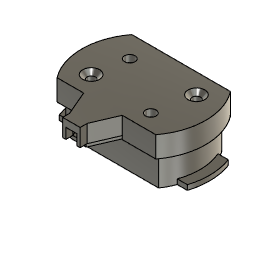
case (Autodesk Fusion 360 design; units mm, degrees)
Autodesk Fusion 360 part; units mm, degrees
sketch "Sketch1" plane through (0, 0, 0) normal (0, 0, 1) x (1, 0, 0)
  circle A0 centre (0, 0) radius 18.75
  line L0 (-17.5873, 6.5) -> (17.5873, 6.5)
  line L1 (-17.5873, -6.5) -> (17.5873, -6.5)
  circle A1 centre (0, 0) radius 16
  line L2 (-17.9252, 5.5) -> (-15.025, 5.5)
  line L3 (15.025, -5.5) -> (17.9252, -5.5)
  line L4 (-13.2288, -9) -> (13.2288, -9)
  line L5 (-13.2288, 9) -> (13.2288, 9)
  dimension "d1" = 37.5
  dimension "d2" = 13
  dimension "d17" = 32
  dimension "d18" = 1
  dimension "d19" = 1
  dimension "d20" = 18
  constraint coincident A0.centre A1.centre
  constraint coincident A0 L0.start
  constraint coincident A0 L0.end
  constraint horizontal L0
  constraint coincident A0 L1.start
  constraint coincident A0 L1.end
  constraint parallel L0 L1
  constraint vertical L0.start L1.start
  constraint concentric A0 A1
  constraint coincident A0 L2.start
  constraint coincident A1 L2.end
  constraint horizontal L2
  constraint coincident A1 L3.start
  constraint coincident A0 L3.end
  constraint parallel L2 L3
  constraint coincident A1 L4.start
  constraint coincident A1 L4.end
  constraint horizontal L4
  constraint coincident A1 L5.start
  constraint coincident A1 L5.end
  constraint parallel L0 L5
  constraint vertical L4.start L5.start
  measures "d1" diameter of A0
  measures "d2" distance of L0.end L1.end
  measures "d17" diameter of A1
  measures "d18" distance of L0 L2
  measures "d19" distance of L1 L3
  measures "d20" distance of L4 L5
extrude "Extrude1" add sketch "Sketch1" along normal blind 1.4 contours A0 L0 A1 L3 | L0 L1 A1 | L0 A1 L5 | A0 L1 A1 L2 | L1 A1 L4 makes body 1
sketch "Sketch2" plane through (0, 0, 0) normal (0, 0, -1) x (1, 0, 0)
  line L0 (-14.6202, 6.5) -> (-17.5873, 6.5)
  circle A0 centre (0, 0) radius 4.75
  circle A1 centre (0, 0) radius 7
  line L1 (4.75, 0) -> (7, 0)
  line L2 (4.4635, -1.6246) -> (6.5778, -2.3941)
  line L3 (4.4635, -1.6246) -> (0, 0)
  arc A2 (17.5873, -6.5) -> (17.9252, 5.5) centre (0, 0) ccw
  line L4 (14.6202, -6.5) -> (17.5873, -6.5)
  arc A3 (-15.025, -5.5) -> (-13.2288, -9) centre (0, 0) ccw
  line L5 (-13.2288, -9) -> (13.2288, -9)
  arc A4 (13.2288, -9) -> (14.6202, -6.5) centre (0, 0) ccw
  line L6 (17.9252, 5.5) -> (15.025, 5.5)
  arc A5 (15.025, 5.5) -> (13.2288, 9) centre (0, 0) ccw
  line L7 (13.2288, 9) -> (-13.2288, 9)
  arc A6 (-13.2288, 9) -> (-14.6202, 6.5) centre (0, 0) ccw
  arc A7 (-17.5873, 6.5) -> (-17.9252, -5.5) centre (0, 0) ccw
  line L8 (-17.9252, -5.5) -> (-15.025, -5.5)
  dimension "d10" = 9.5
  dimension "d11" = 14
  dimension "d12" = 20
  constraint coincident A0.centre A1.centre
  constraint coincident A0 L1.start
  constraint coincident A1 L1.end
  constraint horizontal L1
  constraint coincident A0 L2.start
  constraint coincident A1 L2.end
  constraint horizontal A0.centre L1.start
  constraint parallel L2 L3
  measures "d10" diameter of A0
  measures "d11" diameter of A1
  measures "d12" angle of L1 L2
extrude "Extrude2" add sketch "Sketch2" along normal blind 2.5 contours A0 | A0 A1 L1 L2 picked at (6.2235, -0.4547) bodies 1
sketch "Sketch4" plane through (0, 0, 1.4) normal (0, 0, 1) x (-1, 0, 0)
  arc A0 (13.2288, -9) -> (15.025, -5.5) centre (0, 0) ccw
  line L0 (15.025, -5.5) -> (17.9252, -5.5)
  arc A1 (17.9252, -5.5) -> (17.5873, 6.5) centre (0, 0) ccw
  line L1 (17.5873, 6.5) -> (14.6202, 6.5)
  arc A2 (14.6202, 6.5) -> (13.2288, 9) centre (0, 0) ccw
  line L2 (13.2288, 9) -> (-13.2288, 9)
  arc A3 (-13.2288, 9) -> (-15.025, 5.5) centre (0, 0) ccw
  line L3 (-15.025, 5.5) -> (-17.9252, 5.5)
  arc A4 (-17.9252, 5.5) -> (-17.5873, -6.5) centre (0, 0) ccw
  line L4 (-17.5873, -6.5) -> (-14.6202, -6.5)
  arc A5 (-14.6202, -6.5) -> (-13.2288, -9) centre (0, 0) ccw
  line L5 (-13.2288, -9) -> (13.2288, -9)
  circle A6 centre (0, 0) radius 16
  constraint coincident A0.centre A1.centre
  constraint tangent A0 A6
extrude "Extrude3" add sketch "Sketch4" along normal blind 8 contours A0 A2 L2 A3 A5 L5 A6 bodies 1
sketch "Sketch5" plane through (0, 0, 0) normal (0, 0, -1) x (1, 0, 0)
  line L0 (4.75, 0) -> (7, 0)
  arc A0 (6.5778, -2.3941) -> (7, 0) centre (0, 0) ccw
  line L1 (6.5778, -2.3941) -> (4.4635, -1.6246)
  arc A1 (4.75, 0) -> (4.4635, -1.6246) centre (0, 0) ccw
  arc A2 (-15.025, -5.5) -> (-13.2288, -9) centre (0, 0) ccw
  line L2 (-13.2288, -9) -> (13.2288, -9)
  arc A3 (13.2288, -9) -> (14.6202, -6.5) centre (0, 0) ccw
  line L3 (14.6202, -6.5) -> (17.5873, -6.5)
  arc A4 (17.5873, -6.5) -> (17.9252, 5.5) centre (0, 0) ccw
  line L4 (17.9252, 5.5) -> (15.025, 5.5)
  arc A5 (15.025, 5.5) -> (13.2288, 9) centre (0, 0) ccw
  line L5 (13.2288, 9) -> (-13.2288, 9)
  arc A6 (-13.2288, 9) -> (-14.6202, 6.5) centre (0, 0) ccw
  line L6 (-14.6202, 6.5) -> (-17.5873, 6.5)
  arc A7 (-17.5873, 6.5) -> (-17.9252, -5.5) centre (0, 0) ccw
  line L7 (-17.9252, -5.5) -> (-15.025, -5.5)
  circle A8 centre (-12.5, 0) radius 2.75
  circle A9 centre (12.5, 0) radius 2.75
  line L8 (-12.5, 0) -> (12.5, 0)
  dimension "d23" = 5.5
  dimension "d24" = 5.5
  dimension "d25" = 25
  constraint coincident A8.centre L8.start
  constraint coincident A9.centre L8.end
  constraint midpoint L8 A0.centre
  constraint horizontal L8
  constraint coincident A0.centre A1.centre
  measures "d23" diameter of A8
  measures "d24" diameter of A9
  measures "d25" horizontal distance of A8.centre A9.centre
extrude "Extrude4" cut sketch "Sketch5" against normal blind 10 contours A8 | A9 bodies 1
sketch "Sketch6" plane through (0, 0, 9.4) normal (0, 0, 1) x (-1, 0, 0)
  circle A0 centre (12.5, 0) radius 2.75
  circle A1 centre (-12.5, 0) radius 2.75
  arc A2 (13.2288, -9) -> (13.2288, 9) centre (0, 0) ccw
  line L0 (13.2288, 9) -> (-13.2288, 9)
  arc A3 (-13.2288, 9) -> (-13.2288, -9) centre (0, 0) ccw
  line L1 (-13.2288, -9) -> (13.2288, -9)
  circle A4 centre (12.5, 0) radius 3.1
  circle A5 centre (-12.5, 0) radius 3.1
  dimension "d28" = 6.2
  dimension "d29" = 6.2
  constraint concentric A0 A4
  constraint concentric A1 A5
  measures "d28" diameter of A4
  measures "d29" diameter of A5
extrude "Extrude5" cut sketch "Sketch6" against normal blind 1.5 contours A4 | A5 bodies 1
sketch "Sketch7" plane through (0, 0, 9.4) normal (0, 0, 1) x (-1, 0, 0)
  circle A0 centre (-12.5, 0) radius 3.1
  circle A1 centre (12.5, 0) radius 3.1
  arc A2 (13.2288, -9) -> (13.2288, 9) centre (0, 0) ccw
  line L0 (13.2288, 9) -> (-13.2288, 9)
  arc A3 (-13.2288, 9) -> (-13.2288, -9) centre (0, 0) ccw
  line L1 (-13.2288, -9) -> (13.2288, -9)
  circle A4 centre (10, 5) radius 0.925
  circle A5 centre (-10, -5) radius 0.925
  line L2 (10, 5) -> (-10, -5)
  dimension "d32" = 1.85
  dimension "d33" = 1.85
  dimension "d34" = 20
  dimension "d35" = 10
  constraint coincident A4.centre L2.start
  constraint coincident A5.centre L2.end
  constraint midpoint L2 A2.centre
  constraint coincident A2.centre A3.centre
  measures "d32" diameter of A4
  measures "d33" diameter of A5
  measures "d34" horizontal distance of A4.centre A5.centre
  measures "d35" vertical distance of A4.centre A5.centre
extrude "Extrude6" cut sketch "Sketch7" against normal blind 8 contours A4 | A5 bodies 1
chamfer "Chamfer1" distance 0.3 angle 45 2 edges at (-9.1376, -5.3345, 9.4) (10.8624, 4.6655, 9.4) on bodies 1
copy_body "Body->Comp1" bodies 1 removing the originals makes body 2 in component "bottom"
sketch "Sketch3" plane through (0, 0, 9.4) normal (0, 0, 1) x (-1, 0, 0) in component "top"
  circle A0 centre (10, 5) radius 1.225
  circle A1 centre (-12.5, 0) radius 3.1
  circle A2 centre (12.5, 0) radius 3.1
  arc A3 (13.2288, -9) -> (13.2288, 9) centre (0, 0) ccw
  line L0 (13.2288, 9) -> (-13.2288, 9)
  arc A4 (-13.2288, 9) -> (-13.2288, -9) centre (0, 0) ccw
  line L1 (-13.2288, -9) -> (13.2288, -9)
  circle A5 centre (-10, -5) radius 1.225
  arc A6 (-13.4387, 9.4) -> (-13.4387, -9.4) centre (0, 0) ccw
  line L2 (-13.4387, -9.4) -> (13.4387, -9.4)
  arc A7 (13.4387, -9.4) -> (13.4387, 9.4) centre (0, 0) ccw
  line L3 (13.4387, 9.4) -> (-13.4387, 9.4)
  arc A8 (-14.0748, 10.65) -> (-14.0748, -10.65) centre (0, 0) ccw
  line L4 (-14.0748, -10.65) -> (14.0748, -10.65)
  arc A9 (14.0748, -10.65) -> (14.0748, 10.65) centre (0, 0) ccw
  line L5 (14.0748, 10.65) -> (-14.0748, 10.65)
  dimension "d41" = 0.4
  dimension "d42" = 1.65
extrude "Extrude1'" add sketch "Sketch3" along normal blind 3 and the other way blind 1 separate body contours A8 L4 A9 L5 makes body 3 in component "top"
sketch "Sketch4 (2)" plane through (0, 0, 12.4) normal (0, 0, 1) x (-1, 0, 0) in component "top"
  line L0 (-13.4387, 9.4) -> (13.4387, 9.4)
  arc A0 (13.4387, -9.4) -> (13.4387, 9.4) centre (0, 0) ccw
  line L1 (13.4387, -9.4) -> (-13.4387, -9.4)
  arc A1 (-13.4387, 9.4) -> (-13.4387, -9.4) centre (0, 0) ccw
  line L2 (14.0748, 10.65) -> (-14.0748, 10.65)
  arc A2 (-14.0748, 10.65) -> (-14.0748, -10.65) centre (0, 0) ccw
  line L3 (-14.0748, -10.65) -> (14.0748, -10.65)
  arc A3 (14.0748, -10.65) -> (14.0748, 10.65) centre (0, 0) ccw
extrude "Extrude2'" add sketch "Sketch4 (2)" along normal blind 2 contours L0 A0 L1 A1 | L2 A2 L3 A3 bodies 3 in component "top"
sketch "Sketch5 (2)" plane through (0, 0, 12.4) normal (0, 0, -1) x (1, 0, 0) in component "top"
  arc A0 (13.4387, -9.4) -> (13.4387, 9.4) centre (0, 0) ccw
  line L0 (13.4387, 9.4) -> (-13.4387, 9.4)
  arc A1 (-13.4387, 9.4) -> (-13.4387, -9.4) centre (0, 0) ccw
  line L1 (-13.4387, -9.4) -> (13.4387, -9.4)
  circle A2 centre (-10, 5) radius 1.2
  circle A3 centre (10, -5) radius 1.2
  line L2 (-10, 5) -> (10, -5)
  dimension "d49" = 2.4
  dimension "d50" = 2.4
  dimension "d51" = 20
  dimension "d52" = 10
  constraint coincident A2.centre L2.start
  constraint coincident A3.centre L2.end
  constraint midpoint L2 A0.centre
  constraint coincident A0.centre A1.centre
  measures "d49" diameter of A2
  measures "d50" diameter of A3
  measures "d51" horizontal distance of A2.centre A3.centre
  measures "d52" vertical distance of A2.centre A3.centre
extrude "Extrude3'" cut sketch "Sketch5 (2)" against normal blind 5 contours A2 | A3 bodies 3 in component "top"
sketch "Sketch6 (2)" plane through (0, 0, 12.4) normal (0, 0, -1) x (1, 0, 0) in component "top"
  circle A0 centre (-10, 5) radius 1.2
  circle A1 centre (10, -5) radius 1.2
  arc A2 (13.4387, -9.4) -> (13.4387, 9.4) centre (0, 0) ccw
  line L0 (13.4387, 9.4) -> (-13.4387, 9.4)
  arc A3 (-13.4387, 9.4) -> (-13.4387, -9.4) centre (0, 0) ccw
  line L1 (-13.4387, -9.4) -> (13.4387, -9.4)
  circle A4 centre (-10, 5) radius 1.2
  circle A5 centre (-10, 5) radius 2.7
  circle A6 centre (10, -5) radius 1.2
  circle A7 centre (10, -5) radius 2.7
  circle A8 centre (10, -5) radius 1.2
  dimension "d55" = 1.5
  dimension "d56" = 1.5
  constraint concentric A0 A4
  constraint concentric A0 A5
  constraint concentric A1 A6
  constraint concentric A6 A7
  constraint equal A0 A4
  constraint equal A6 A8
  measures "d55" distance of A4 A5
  measures "d56" distance of A6 A7
extrude "Extrude4'" add sketch "Sketch6 (2)" along normal blind 2 contours A5 | A7 bodies 3 in component "top"
chamfer "Chamfer1'" distance 1.2 angle 45 2 edges at (-11.1188, -4.5661, 14.4) (8.8812, 5.4339, 14.4) on bodies 3 in component "top"
sketch "Sketch8" plane through (0, 0, 14.4) normal (0, 0, 1) x (-1, 0, 0)
  circle A0 centre (10, 5) radius 2.4
  arc A1 (14.0748, -10.65) -> (14.0748, 10.65) centre (0, 0) ccw
  line L0 (14.0748, 10.65) -> (-14.0748, 10.65)
  arc A2 (-14.0748, 10.65) -> (-14.0748, -10.65) centre (0, 0) ccw
  line L1 (-14.0748, -10.65) -> (14.0748, -10.65)
  circle A3 centre (-10, -5) radius 2.4
  line L2 (6.5, 10.65) -> (3.5, 17.65)
  line L3 (3.5, 17.65) -> (-1.5, 17.65)
  line L4 (-1.5, 17.65) -> (-4.5, 10.65)
  point P0 (1, 17.65)
  dimension "d60" = 7
  dimension "d61" = 3
  dimension "d62" = 5
  dimension "d63" = 3
  dimension "d64" = 9
  constraint coincident L0 L2.start
  constraint parallel L0 L3
  constraint coincident L0 L4.end
  constraint midpoint L3 P0
  measures "d60" distance of L0 L3
  measures "d61" horizontal distance of L3.end L4.end
  measures "d62" distance of L2.end L3.end
  measures "d63" horizontal distance of L2.start L2.end
  measures "d64" horizontal distance of A0.centre P0
extrude "Extrude5'" add sketch "Sketch8" against normal blind 2 contours L0 L2 L3 L4 bodies 3 in component "top"
sketch "Sketch9" plane through (0, 0, 8.4) normal (0, 0, -1) x (1, 0, 0)
  line L0 (-13.4387, 9.4) -> (13.4387, 9.4)
  arc A0 (13.4387, -9.4) -> (13.4387, 9.4) centre (0, 0) ccw
  line L1 (13.4387, -9.4) -> (-13.4387, -9.4)
  arc A1 (-13.4387, 9.4) -> (-13.4387, -9.4) centre (0, 0) ccw
  line L2 (14.0748, 10.65) -> (-14.0748, 10.65)
  arc A2 (-14.0748, 10.65) -> (-14.0748, -10.65) centre (0, 0) ccw
  line L3 (-14.0748, -10.65) -> (14.0748, -10.65)
  arc A3 (14.0748, -10.65) -> (14.0748, 10.65) centre (0, 0) ccw
  line L4 (-6.5, 10.65) -> (-7.0357, 9.4)
  line L5 (4.5, 10.65) -> (5.0357, 9.4)
  line L6 (-3.5, 17.65) -> (-6.5, 10.65)
  line L7 (4.5, 10.65) -> (1.5, 17.65)
  constraint coincident L2 L4.start
  constraint coincident L0 L4.end
  constraint coincident L2 L5.start
  constraint coincident L0 L5.end
  constraint parallel L4 L6
  constraint parallel L5 L7
  constraint coincident L4.start L6.end
  constraint coincident L5.start L7.start
extrude "Extrude6'" cut sketch "Sketch9" against normal blind 4 contours L0 L2 L4 L5 bodies 3 in component "top"
sketch "Sketch10" plane through (0, 0, 12.4) normal (0, 0, -1) x (1, 0, 0)
  circle A0 centre (-10, 5) radius 2.7
  circle A1 centre (10, -5) radius 2.7
  line L0 (-3.5, 17.65) -> (-6.5, 10.65)
  line L1 (-6.5, 10.65) -> (-7.0357, 9.4)
  line L2 (-7.0357, 9.4) -> (-13.4387, 9.4)
  arc A2 (-13.4387, 9.4) -> (-13.4387, -9.4) centre (0, 0) ccw
  line L3 (-13.4387, -9.4) -> (13.4387, -9.4)
  arc A3 (13.4387, -9.4) -> (13.4387, 9.4) centre (0, 0) ccw
  line L4 (13.4387, 9.4) -> (5.0357, 9.4)
  line L5 (5.0357, 9.4) -> (4.5, 10.65)
  line L6 (4.5, 10.65) -> (1.5, 17.65)
  line L7 (1.5, 17.65) -> (-3.5, 17.65)
  line L8 (-7.0357, 9.4) -> (-6.1109, 9.4)
  line L9 (-6.1109, 9.4) -> (-2.5752, 17.65)
  line L10 (0.5752, 17.65) -> (4.1109, 9.4)
  line L11 (4.1109, 9.4) -> (5.0357, 9.4)
  dimension "d69" = 0.85
  dimension "d70" = 0.85
  constraint coincident L1.end L2.start
  constraint parallel L2 L8
  constraint coincident L7 L9.end
  constraint coincident L7 L10.start
  constraint coincident L4.end L5.start
  constraint parallel L4 L11
  constraint parallel L0 L9
  constraint parallel L6 L10
  measures "d69" distance of L0 L9
  measures "d70" distance of L6 L10
extrude "Extrude7" add sketch "Sketch10" along normal blind 3 contours L0 L1 L7 L8 L9 | L5 L6 L7 L10 L11 bodies 3 in component "top"
extrude "Extrude8" add 1 faces at (-0.4749, -17.65, 13.7333) along direction (0, -1, 0) blind 2 on bodies 3 bodies 3 in component "top"
sketch "Sketch11" plane through (0, 0, 14.4) normal (0, 0, 1) x (-1, 0, 0)
  circle A0 centre (10, 5) radius 2.4
  arc A1 (14.0748, -10.65) -> (14.0748, 10.65) centre (0, 0) ccw
  line L0 (14.0748, 10.65) -> (6.5, 10.65)
  line L1 (6.5, 10.65) -> (3.5, 17.65)
  line L2 (3.5, 17.65) -> (3.5, 19.65)
  line L3 (3.5, 19.65) -> (-1.5, 19.65)
  line L4 (-1.5, 19.65) -> (-1.5, 17.65)
  line L5 (-1.5, 17.65) -> (-4.5, 10.65)
  line L6 (-4.5, 10.65) -> (-14.0748, 10.65)
  arc A2 (-14.0748, 10.65) -> (-14.0748, -10.65) centre (0, 0) ccw
  line L7 (-14.0748, -10.65) -> (14.0748, -10.65)
  circle A3 centre (-10, -5) radius 2.4
  circle A4 centre (8.4, -4.4) radius 1.5
  circle A5 centre (-8, 6) radius 1.5
  circle A6 centre (10, 5) radius 1.2
  circle A7 centre (-10, -5) radius 1.2
  dimension "d75" = 3
  dimension "d76" = 3
  dimension "d77" = 1.6
  dimension "d78" = 0.6
  dimension "d79" = 2
  dimension "d80" = 1
  measures "d75" diameter of A4
  measures "d76" diameter of A5
  measures "d77" horizontal distance of A4.centre A0.centre
  measures "d78" vertical distance of A4.centre A3.centre
  measures "d79" horizontal distance of A5.centre A3.centre
  measures "d80" vertical distance of A5.centre A0.centre
extrude "Extrude9" cut sketch "Sketch11" against normal blind 2 contours A4 | A5 bodies 3 in component "top"
sketch "Sketch12" plane through (0, 0, 9.4) normal (0, 0, 1) x (-1, 0, 0)
  circle A0 centre (10, 5) radius 1.225
  circle A1 centre (-12.5, 0) radius 3.1
  circle A2 centre (12.5, 0) radius 3.1
  arc A3 (13.2288, -9) -> (13.2288, 9) centre (0, 0) ccw
  line L0 (13.2288, 9) -> (-13.2288, 9)
  arc A4 (-13.2288, 9) -> (-13.2288, -9) centre (0, 0) ccw
  line L1 (-13.2288, -9) -> (13.2288, -9)
  circle A5 centre (-10, -5) radius 1.225
  line L2 (6.9352, 9) -> (3.228, 17.65)
  line L3 (3.228, 17.65) -> (-1.228, 17.65)
  line L4 (-1.228, 17.65) -> (-4.9352, 9)
  line L5 (3.5, 17.65) -> (6.5, 10.65)
  line L6 (-4.5, 10.65) -> (-1.5, 17.65)
  point P0 (2.5752, 17.65)
  dimension "d93" = 0.25
  dimension "d94" = 0.25
  constraint coincident L0 L2.start
  constraint parallel L0 L3
  constraint coincident L0 L4.end
  constraint parallel L2 L5
  constraint parallel L4 L6
  constraint coincident L3 P0
  measures "d93" distance of L4 L6
  measures "d94" distance of L2 L5
extrude "Extrude3''" add sketch "Sketch12" against normal blind 1 contours L0 L2 L3 L4 bodies 2 in component "bottom"
component "top" placed x (1, 0, 0) y (0, 1, 0) z (0, 0, 1) at (0, 0, 0)
component "bottom" placed x (1, 0, 0) y (0, 1, 0) z (0, 0, 1) at (0, 0, 0)
equation "bottom_thickness = 1.4 mm"
equation "d8 = bottom_thickness"
equation "d42 = 1.25 mm + 0.4 mm"
